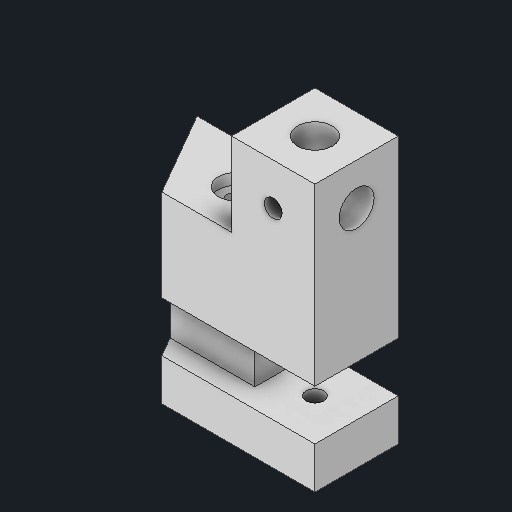
# Autodesk Inventor part: A Idler
Saved by Autodesk Inventor 2025.1 (Build 291241020, 241B)
## iProperties
Created: 2025-04-15
Part Number: A Idler
Material: Generic
Document SubType Name: Modeling
Designer: Joshua Eah
Density: 1 g/cm^3
Appearance: Default
Author: Joshua Eah
Autodesk Inventor part; units mm, degrees
ref_plane "YZ Plane" through (0, 0, 0) normal (1, 0, 0) x (0, 1, 0)
ref_plane "XZ Plane" through (0, 0, 0) normal (0, 1, 0) x (-1, 0, 0)
ref_plane "XY Plane" through (0, 0, 0) normal (0, 0, 1) x (1, 0, 0)
sketch "Sketch1" plane through (0, 0, 0) normal (0, 1, 0) x (-1, 0, 0)
  line L0 (0, 0) -> (36.2103, 0)
  line L1 (36.2103, 0) -> (36.2103, -15)
  line L2 (36.2103, -15) -> (0, -15)
  line L3 (0, -15) -> (0, 0)
  dimension "d0" = 36.2103
  dimension "d1" = 15
  constraints: 8 end point, 2 parallel, 1 horizontal, 1 perpendicular
  measures "d0" distance of L1.end L2.end
  measures "d1" distance of L0.end L1.end
extrude "Extrusion1" add sketch "Sketch1" along normal blind 48
sketch "Sketch2" plane through (-36.2103, 0, 0) normal (0, 0, 1) x (1, 0, 0)
  line L0 (0, 0) -> (36.2103, 0) projected
  line L1 (36.2103, 0) -> (36.2103, 48) projected
  line L2 (0, 48) -> (36.2103, 48) projected
  line L3 (0, 0) -> (0, 48) projected
  line L4 (0, 7.5) -> (36.2103, 7.5)
  line L5 (36.2103, 7.5) -> (36.2103, 16.5)
  line L6 (36.2103, 16.5) -> (0, 16.5)
  line L7 (0, 16.5) -> (0, 7.5)
  point P0 (0, 16.5)
  dimension "d10" = 9
  dimension "d11" = 7.5
  constraints: 8 end point, 2 parallel, 2 point on line, 1 horizontal, 1 perpendicular
  measures "d10" distance between parallel lines of L4 L6
  measures "d11" distance between parallel lines of L0 L4
extrude "Extrusion2" cut sketch "Sketch2" against normal blind 3.5 contours L3 L6 L1 L4
sketch "Sketch3" plane through (0, 0, -15) normal (0, 0, -1) x (-1, 0, 0)
  line L0 (0, 0) -> (36.2103, 0) projected
  line L1 (36.2103, 0) -> (36.2103, 48) projected
  line L2 (0, 48) -> (36.2103, 48) projected
  line L3 (0, 0) -> (0, 48) projected
  line L4 (0, 7.5) -> (36.2103, 7.5)
  line L5 (36.2103, 7.5) -> (36.2103, 16.5)
  line L6 (36.2103, 16.5) -> (0, 16.5)
  line L7 (0, 16.5) -> (0, 7.5)
  point P0 (0, 16.5)
  dimension "d14" = 7.5
  dimension "d15" = 9
  constraints: 8 end point, 2 parallel, 2 point on line, 1 horizontal, 1 perpendicular
  measures "d14" distance between parallel lines of L0 L4
  measures "d15" distance between parallel lines of L4 L6
extrude "Extrusion3" cut sketch "Sketch3" against normal blind 3.5 contours L3 L6 L1 L4
sketch "Sketch4" plane through (0, 0, 0) normal (1, 0, 0) x (0, 0, -1)
  line L0 (15, 7.5) -> (11.5, 7.5) projected
  line L1 (11.5, 7.5) -> (11.5, 16.5) projected
  line L2 (11.5, 16.5) -> (15, 16.5) projected
  line L3 (15, 16.5) -> (15, 48) projected
  line L4 (0, 48) -> (15, 48) projected
  line L5 (0, 16.5) -> (0, 48) projected
  line L6 (0, 16.5) -> (3.5, 16.5) projected
  line L7 (3.5, 16.5) -> (3.5, 7.5) projected
  line L8 (3.5, 7.5) -> (0, 7.5) projected
  line L9 (0, 0) -> (0, 7.5) projected
  line L10 (0, 0) -> (15, 0) projected
  line L11 (15, 0) -> (15, 7.5) projected
  line L12 (3.5, 7.5) -> (11.5, 7.5)
  line L13 (11.5, 7.5) -> (11.5, 16.5)
  line L14 (11.5, 16.5) -> (3.5, 16.5)
  line L15 (3.5, 16.5) -> (3.5, 7.5)
  constraints: 8 end point, 2 parallel, 1 horizontal, 1 perpendicular
extrude "Extrusion4" cut sketch "Sketch4" against normal blind 14.3 contours L12 L7 L14 L1
sketch "Sketch5" plane through (0, 48, 0) normal (0, 1, 0) x (1, 0, 0)
  line L0 (0, 15) -> (-36.2103, 15) projected
  line L1 (-36.2103, 15) -> (-36.2103, 0) projected
  line L2 (-36.2103, 0) -> (0, 0) projected
  line L3 (0, 0) -> (0, 15) projected
  line L4 (-36.2103, 0) -> (0, 0) projected
  line L5 (-15, 0) -> (-36.2103, 0)
  line L6 (-36.2103, 0) -> (-36.2103, 15)
  line L7 (-36.2103, 15) -> (-15.0001, 15)
  line L8 (-15.0001, 15) -> (-15, 0)
  point P0 (-15.0001, 15)
  dimension "d20" = 21.2102
  constraints: 8 end point, 2 parallel, 1 horizontal, 1 perpendicular, 1 point on line
  measures "d20" distance between parallel lines of L1 L8
extrude "Extrusion5" cut sketch "Sketch5" against normal blind 15 contours L8 L2 L1 L0
sketch "Sketch6" plane through (0, 33, 0) normal (0, 1, 0) x (1, 0, 0)
  line L0 (-36.2103, 15) -> (-15.0001, 15) projected
  line L1 (-36.2103, 0) -> (-36.2103, 15) projected
  line L2 (-15, 0) -> (-36.2103, 0) projected
  line L3 (-15.0001, 15) -> (-15, 0) projected
  circle A0 centre (-21.7, 7.5) radius 1.3741
  line L4 (0, 0) -> (0, 15) projected
  dimension "d23" = 7.5
  dimension "d24" = 21.7
  constraints: 1 centre point
  measures "d23" distance from line of A0.centre L2
  measures "d24" distance from line of L4 A0.centre
hole "Hole1" at (-21.7, 33, -7.5) direction (0, -1, 0) diameter 3.2004 end through all counterbore diameter 6.2992 counterbore depth 2 clearance for "Oval Head Machine Screw" size "M3" standard "Ansi Metric M Profile"
sketch "Sketch7" plane through (0, 48, 0) normal (0, 1, 0) x (1, 0, 0)
  line L0 (-15.0001, 15) -> (-15, 0) projected
  line L1 (-15, 0) -> (0, 0) projected
  line L2 (0, 0) -> (0, 15) projected
  line L3 (0, 15) -> (-15.0001, 15) projected
  circle A0 centre (-7.5, 7.5) radius 1.6
  dimension "d32" = 3.2
  dimension "d33" = 7.5
  dimension "d34" = 7.5
  constraints: 1 centre point
  measures "d32" diameter of A0
  measures "d33" distance from line of L1 A0.centre
  measures "d34" distance from line of L2 A0.centre
hole "Hole2" at (-7.5, 48, -7.5) direction (0, -1, 0) diameter 3.2004 end through all counterbore diameter 6.2992 counterbore depth 17 clearance for "Oval Head Machine Screw" size "M3" standard "Ansi Metric M Profile"
sketch "Sketch8" plane through (0, 48, 0) normal (1, 0, 0) x (0, 0, -1)
  line L0 (0, -31.5) -> (15, -31.5) projected
  line L1 (15, -31.5) -> (15, 0) projected
  line L2 (0, 0) -> (15, 0) projected
  line L3 (0, -31.5) -> (0, 0) projected
  circle A0 centre (7.5, -7.5) radius 1.6
  point P0 (0, -48)
  dimension "d42" = 3.2
  dimension "d43" = 7.5
  dimension "d44" = 7.5
  constraints: 1 centre point
  measures "d42" diameter of A0
  measures "d43" distance from line of L2 A0.centre
  measures "d44" distance from line of L3 A0.centre
hole "Hole3" at (0, 40.5, -7.5) direction (-1, 0, 0) diameter 3.2004 end through all counterbore diameter 6.2992 counterbore depth 12 clearance for "Oval Head Machine Screw" size "M3" standard "Ansi Metric M Profile"
sketch "Sketch10" plane through (0, 16.5, -15) normal (0, 0, -1) x (-1, 0, 0)
  line L0 (36.2103, 16.5) -> (15.0001, 16.5) projected
  line L1 (15.0001, 16.5) -> (15.0001, 31.5) projected
  line L2 (0, 31.5) -> (15.0001, 31.5) projected
  line L3 (0, 0) -> (0, 31.5) projected
  line L4 (0, 0) -> (36.2103, 0) projected
  line L5 (36.2103, 0) -> (36.2103, 16.5) projected
  circle A0 centre (7.5, 24) radius 1.6
  point P0 (0, -16.5)
  dimension "d62" = 3.2
  dimension "d63" = 7.5
  dimension "d64" = 7.5
  constraints: 1 centre point
  measures "d62" diameter of A0
  measures "d63" distance from line of A0.centre L2
  measures "d64" distance from line of A0.centre L3
hole "Hole5" at (-7.5, 40.5, -15) direction (0, 0, 1) diameter 3.2004 end through all counterbore diameter 6.2992 counterbore depth 12 clearance for "Oval Head Machine Screw" size "M3" standard "Ansi Metric M Profile"
chamfer "Chamfer2" distance 15 angle 30 2 edges at (-36.2103, 24.75, 0) (-36.2103, 3.75, 0) measured on face at (-36.2103, 3.75, -0.5) measured on face at (-36.2103, 24.75, -0.5)
body "Solid1"
